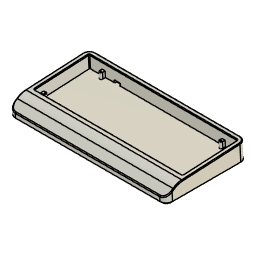
SK-Vault 37 (Autodesk Fusion 360 design; units mm, degrees)
Autodesk Fusion 360 part; units mm, degrees
sketch "Base Plane Sketch" plane through (0, 0, 0) normal (0, 0, 1) x (1, 0, 0)
  line L0 (0, 0) -> (209.55, 0) construction
  line L1 (209.55, 0) -> (209.55, -57.15) construction
  line L2 (28.575, -76.2) -> (180.975, -76.2) construction
  line L3 (-7.5, 7.5) -> (217.05, 7.5)
  line L4 (217.05, 7.5) -> (217.05, -64.65)
  line L5 (21.075, -83.7) -> (188.475, -83.7)
  line L6 (-7.5, 7.5) -> (-7.5, -64.65)
  line L7 (-7.5, -64.65) -> (-7.5, -83.7)
  line L8 (-7.5, -83.7) -> (21.075, -83.7)
  line L9 (188.475, -83.7) -> (217.05, -83.7)
  line L10 (217.05, -83.7) -> (217.05, -64.65)
  line L11 (-7.5, -83.7) -> (-7.5, -90.7)
  line L12 (-7.5, -90.7) -> (217.05, -90.7)
  line L13 (217.05, -90.7) -> (217.05, -83.7)
  line L14 (-1.075, 1.075) -> (-1.075, -57.15)
  line L15 (27.5, -77.275) -> (182.05, -77.275)
  line L16 (210.625, 1.075) -> (210.625, -58.225)
  line L17 (0, 1.075) -> (210.625, 1.075)
  line L18 (-1.075, -57.15) -> (-1.075, -58.225)
  line L19 (0, 1.075) -> (-1.075, 1.075)
  line L20 (209.55, 0) -> (190.5, 0) construction
  line L21 (190.5, 0) -> (190.5, -19.05) construction
  line L22 (190.5, -19.05) -> (209.55, -19.05) construction
  line L23 (209.55, -19.05) -> (209.55, 0) construction
  line L24 (190.5, -9.525) -> (209.55, -9.525) construction
  line L25 (200.025, -19.05) -> (200.025, 0) construction
  circle A0 centre (19.05, -2.525) radius 2.25
  line L26 (19.05, -2.525) -> (190.5, -2.525) construction
  circle A1 centre (190.5, -2.525) radius 2.25
  line L27 (21.3, -2.525) -> (21.3, 1.075)
  line L28 (192.75, -2.525) -> (192.75, 1.075)
  line L29 (188.25, -2.525) -> (188.25, 1.075)
  line L30 (16.8193, -2.2307) -> (16.8193, 1.075)
  line L31 (-1.075, -58.225) -> (-1.075, -77.275)
  line L32 (-1.075, -77.275) -> (27.5, -77.275)
  line L33 (210.625, -58.225) -> (210.625, -77.275)
  line L34 (210.625, -77.275) -> (182.05, -77.275)
  line L35 (-0.125, 0.125) -> (209.675, 0.125) construction
  line L36 (209.675, 0.125) -> (209.675, -76.325) construction
  line L37 (-0.125, -76.325) -> (-0.125, 0.125) construction
  line L38 (47.5, -76.325) -> (47.5, -57.275) construction
  line L39 (47.5, -57.275) -> (28.7, -57.275) construction
  line L40 (28.7, -57.275) -> (28.7, -76.325) construction
  line L41 (180.85, -76.325) -> (180.85, -57.275) construction
  line L42 (180.85, -57.275) -> (162.05, -57.275) construction
  line L43 (162.05, -57.275) -> (162.05, -76.325) construction
  circle A2 centre (19.05, -2.525) radius 1 construction
  circle A3 centre (190.5, -2.525) radius 1 construction
  circle A4 centre (207.284, -66.384) radius 1 construction
  circle A5 centre (2.266, -66.384) radius 1 construction
  line L44 (28.7, -76.325) -> (-0.125, -76.325) construction
  line L45 (209.675, -76.325) -> (180.85, -76.325) construction
  line L46 (162.05, -76.325) -> (47.5, -76.325) construction
  line L47 (179.9, -76.325) -> (179.9, -77.275)
  line L48 (163, -76.325) -> (163, -77.275)
  line L49 (29.65, -76.325) -> (29.65, -77.275)
  line L50 (46.55, -76.325) -> (46.55, -77.275)
  circle A6 centre (2.266, -66.384) radius 2.25
  circle A7 centre (207.284, -66.384) radius 2.25
  line L51 (207.284, -64.134) -> (210.625, -64.134)
  line L52 (207.284, -68.634) -> (210.625, -68.634)
  line L53 (2.266, -64.134) -> (-1.075, -64.134)
  line L54 (2.266, -68.634) -> (-1.075, -68.634)
  point P0 (9.525, -9.525)
  point P1 (9.525, -47.625)
  dimension "d1" = 209.55
  dimension "d2" = 57.15
  dimension "d39" = 7
  dimension "d117" = 19.05
  dimension "d118" = 19.05
  dimension "d122" = 4.5
  dimension "d180" = 209.8
  dimension "d181" = 76.45
  dimension "d182" = 19.05
  dimension "d183" = 18.8
  dimension "d184" = 28.825
  dimension "d185" = 18.8
  dimension "d186" = 19.05
  dimension "d187" = 28.825
  dimension "d188" = 2
  dimension "d189" = 2
  dimension "d190" = 2
  dimension "d191" = 2
  dimension "d192" = 19.175
  dimension "d193" = 2.65
  dimension "d194" = 2.65
  dimension "d195" = 19.175
  dimension "d196" = 2.391
  dimension "d197" = 9.941
  dimension "d198" = 9.941
  dimension "d199" = 2.391
  dimension "d202" = 4.5
  dimension "d203" = 4.5
  constraint coincident L0.start origin
  constraint horizontal L0
  constraint perpendicular L0 L1
  constraint perpendicular L5 L7
  constraint perpendicular L4 L9
  constraint vertical L11
  constraint perpendicular L10 L12
  constraint perpendicular L9 L13
  constraint perpendicular L14 L19
  constraint horizontal L20
  constraint vertical L21
  constraint horizontal L22
  constraint vertical L23
  constraint midpoint L21 L24.start
  constraint midpoint L23 L24.end
  constraint midpoint L22 L25.start
  constraint midpoint L20 L25.end
  constraint coincident A0.centre L26.start
  constraint coincident L21 L26.end
  constraint perpendicular L21 L26
  constraint coincident L26.end A1.centre
  constraint coincident A0 L27.start
  constraint coincident L26 L27.start
  constraint coincident L17 L27.end
  constraint tangent A0 L27
  constraint coincident A1 L28.start
  constraint coincident L17 L28.end
  constraint tangent A1 L28
  constraint perpendicular L17 L28
  constraint coincident L26 L29.start
  constraint coincident A1 L29.start
  constraint coincident L17 L29.end
  constraint tangent A1 L29
  constraint coincident A0 L30.start
  constraint coincident L17 L30.end
  constraint perpendicular L17 L30
  constraint equal A0 A1
  constraint perpendicular L15 L31
  constraint perpendicular L31 L32
  constraint perpendicular L15 L33
  constraint horizontal L35
  constraint vertical L36
  constraint horizontal L45
  constraint vertical L37
  constraint vertical L38
  constraint horizontal L39
  constraint vertical L40
  constraint coincident L40.end L45
  constraint vertical L41
  constraint horizontal L42
  constraint vertical L43
  constraint coincident L43.end L45
  constraint collinear L44 L45
  constraint collinear L45 L46
  constraint coincident L15 L47.end
  constraint perpendicular L15 L47
  constraint coincident L15 L48.end
  constraint perpendicular L15 L48
  constraint coincident L15 L49.end
  constraint perpendicular L15 L49
  constraint coincident L15 L50.end
  constraint perpendicular L15 L50
  constraint concentric A5 A6
  constraint concentric A4 A7
  constraint coincident A7 L51.start
  constraint coincident L33 L51.end
  constraint tangent A7 L51
  constraint perpendicular L33 L51
  constraint coincident A7 L52.start
  constraint coincident L33 L52.end
  constraint tangent A7 L52
  constraint perpendicular L33 L52
  constraint coincident A6 L53.start
  constraint coincident L31 L53.end
  constraint tangent A6 L53
  constraint perpendicular L31 L53
  constraint coincident A6 L54.start
  constraint coincident L31 L54.end
  constraint tangent A6 L54
  constraint perpendicular L31 L54
  measures "d1" distance of L0.start L0.end
  measures "d2" distance of L0.end L1.end
  measures "d39" distance of L7.end L11.end
  measures "d117" distance of L0.end L20.end
  measures "d118" distance of L0.end L22.end
  measures "d122" diameter of A0
  measures "d180" distance of L35.start L35.end
  measures "d181" distance of L35.start L37.start
  measures "d182" distance of L40.end L39.end
  measures "d183" distance of L38.end L39.end
  measures "d184" distance of L37 L40
  measures "d185" distance of L43.end L41.start
  measures "d186" distance of L43.end L42.end
  measures "d187" distance of L36 L41
  measures "d188" diameter of A2
  measures "d189" diameter of A3
  measures "d190" diameter of A4
  measures "d191" diameter of A5
  measures "d192" distance of L37 A0.centre
  measures "d193" distance of L35 A0.centre
  measures "d194" distance of L35 L26.end
  measures "d195" distance of L36 L26.end
  measures "d196" distance of L37 A5.centre
  measures "d197" distance of A5.centre L45
  measures "d198" distance of A4.centre L45
  measures "d199" distance of L36 A4.centre
  measures "d202" diameter of A6
  measures "d203" diameter of A7
extrude "External Base Extrude" add sketch "Base Plane Sketch" along normal blind 21.06
extrude "Internal Base Extrude" add sketch "Base Plane Sketch" 1 faces at (85.3667, -86.225, 0) along normal blind 3 contours L14 L15 L16 L17 L18 L19 A0 A1 L27 L28 L29 L30 L31 L32 L33 L34 A6 A7 L51 L52 L53 L54 | L17 A0 L27 L30 | L31 A6 L53 L54 | A0 | A6 | L17 A1 L28 L29 | A1 | L33 A7 L51 L52 | A7
sketch "Side Plane Sketch" plane through (-7.5, 0, 0) normal (-1, 0, 0) x (0, -1, 0)
  line L0 (90.7, 0) -> (90.7, 21.06)
  line L1 (90.7, 21.06) -> (-7.5, 21.06)
  line L2 (-7.5, 21.06) -> (-7.5, 0)
  line L3 (-7.5, 0) -> (90.7, 0)
  line L4 (90.7, 21.06) -> (107.8598, 10)
  line L5 (107.8598, 10) -> (107.8598, 0)
  line L6 (107.8598, 0) -> (90.7, 0)
  dimension "d149" = 10
  constraint coincident L0.end L1.start
  constraint perpendicular L3 L5
  constraint coincident L0.start L3.end
  constraint perpendicular L0 L6
  measures "d149" distance of L4.end L5.end
extrude "Wrist Wrest Extrude" add sketch "Side Plane Sketch" against normal up to surface (224.55 mm away) contours L0 L4 L5 L6
fillet "Outside Vertical Fillets" radius 9 4 edges at (-7.5, -107.8598, 5) (217.05, -107.8598, 5) (217.05, 7.5, 10.53) (-7.5, 7.5, 10.53)
fillet "Wrist Wrest Angle Fillet" radius 23.5 1 edges at (104.775, -90.7, 21.06)
fillet "Inside Case Vertical Fillets" radius 1 4 edges at (210.625, 1.075, 12.03) (210.625, -77.275, 12.03) (-1.075, -77.275, 12.03) (-1.075, 1.075, 12.03)
chamfer "Top Outside Edge Chamfer" distance 1 angle 45 12 edges at (-7.5, -42.6415, 21.06) (-7.5, -90.4185, 20.1037) (-7.5, -97.6869, 16.5567) (-4.864, -105.2238, 11.699) (104.775, -107.8598, 10) (214.414, -105.2238, 11.699) (217.05, -97.6869, 16.5567) (217.05, -90.4185, 20.1037) (217.05, -42.6415, 21.06) (214.414, 4.864, 21.06) (104.775, 7.5, 21.06) (-4.864, 4.864, 21.06)
chamfer "Top Inside Edge Chamfer" distance 1 angle 45 8 edges at (210.625, -38.1, 21.06) (210.3321, -76.9821, 21.06) (104.775, -77.275, 21.06) (-0.7821, -76.9821, 21.06) (-1.075, -38.1, 21.06) (-0.7821, 0.7821, 21.06) (104.775, 1.075, 21.06) (210.3321, 0.7821, 21.06)
sketch "USB C Hole Internal" plane through (0, 1.075, 0) normal (0, -1, 0) x (1, 0, 0)
  line L0 (193, 10.9) -> (193, 3)
  line L1 (193, 3) -> (209.05, 3)
  line L2 (209.05, 3) -> (209.05, 17.06)
  line L3 (209.05, 17.06) -> (0.5, 17.06)
  line L4 (0.5, 17.06) -> (0.5, 3)
  line L5 (0.5, 3) -> (16.55, 3)
  line L6 (16.55, 3) -> (16.55, 10.9)
  line L7 (16.55, 10.9) -> (21.55, 10.9)
  line L8 (21.55, 10.9) -> (21.55, 3)
  line L9 (21.55, 3) -> (188, 3)
  line L10 (188, 3) -> (188, 10.9)
  line L11 (188, 10.9) -> (193, 10.9)
  line L12 (0.5, 3) -> (0, 3) construction
  line L13 (34.925, 3) -> (38.1, 3) construction
  line L14 (41.275, 6.66) -> (34.925, 6.66)
  line L15 (33.375, 5.11) -> (33.375, 4.55)
  line L16 (33.375, 3) -> (41.275, 3)
  line L17 (42.825, 4.55) -> (42.825, 5.11)
  line L18 (42.825, 6.66) -> (33.375, 3) construction
  line L19 (33.375, 6.66) -> (42.825, 3) construction
  arc A0 (34.925, 6.66) -> (33.375, 5.11) centre (34.925, 5.11) ccw
  arc A1 (42.825, 5.11) -> (41.275, 6.66) centre (41.275, 5.11) ccw
  arc A2 (41.275, 3) -> (42.825, 4.55) centre (41.275, 4.55) ccw
  arc A3 (33.375, 4.55) -> (34.925, 3) centre (34.925, 4.55) ccw
  line L20 (209.625, 20.06) -> (-0.075, 20.06)
  line L21 (-0.075, 20.06) -> (-0.075, 3)
  line L22 (-0.075, 3) -> (209.625, 3)
  line L23 (209.625, 3) -> (209.625, 20.06)
  point P0 (38.1, 4.83)
  dimension "d75" = 0.5
  dimension "d79" = 1.55
  dimension "d80" = 9.45
  dimension "d82" = 38.1
  dimension "d83" = 3.66
  constraint coincident L4.end L5.start
  constraint perpendicular L4 L12
  constraint parallel L5 L13
  constraint horizontal L14
  constraint perpendicular L14 L15
  constraint parallel L14 L16
  constraint parallel L15 L17
  constraint coincident L18 P0
  constraint coincident L19 P0
  constraint coincident L19.start L15
  constraint coincident L19.start L14
  constraint tangent L15 A0
  constraint tangent L14 A0
  constraint coincident L18.start L14
  constraint coincident L18.start L17
  constraint tangent L14 A1
  constraint tangent L17 A1
  constraint equal A0 A1
  constraint coincident L19.end L17
  constraint coincident L19.end L16
  constraint tangent L17 A2
  constraint tangent L16 A2
  constraint equal A0 A2
  constraint coincident L12.end L13
  constraint coincident L16.start L15
  constraint tangent L13 A3
  constraint tangent L15 A3
  constraint equal A0 A3
  measures "d75" distance of L4.end L12.end
  measures "d79" radius of A0
  measures "d80" distance of L15 L17
  measures "d82" distance of L12.end L13.end
  measures "d83" distance of L13.end L14
extrude "Internal USB C Extrude Cut" cut sketch "USB C Hole Internal" against normal blind 24 contours L9 L14 L15 L16 L17 A0 A1 A2 A3 L22
sketch "USB C Hole External" plane through (0, 7.5, 0) normal (0, 1, 0) x (-1, 0, 0)
  arc A0 (-42.825, 4.55) -> (-41.275, 3) centre (-41.275, 4.55) ccw
  line L0 (-42.825, 4.55) -> (-42.825, 5.11)
  arc A1 (-41.275, 6.66) -> (-42.825, 5.11) centre (-41.275, 5.11) ccw
  line L1 (-41.275, 6.66) -> (-34.925, 6.66)
  arc A2 (-33.375, 5.11) -> (-34.925, 6.66) centre (-34.925, 5.11) ccw
  line L2 (-33.375, 5.11) -> (-33.375, 4.55)
  arc A3 (-34.925, 3) -> (-33.375, 4.55) centre (-34.925, 4.55) ccw
  line L3 (-42.825, 4.83) -> (-33.375, 4.83) construction
  line L4 (-38.1, 6.66) -> (-38.1, 3) construction
  line L5 (-34.925, 8.91) -> (-41.275, 8.91)
  line L6 (-45.075, 5.11) -> (-45.075, 4.55)
  line L7 (-41.275, 0.75) -> (-34.925, 0.75)
  line L8 (-31.125, 4.55) -> (-31.125, 5.11)
  line L9 (-31.125, 8.91) -> (-45.075, 0.75) construction
  line L10 (-45.075, 8.91) -> (-31.125, 0.75) construction
  arc A4 (-41.275, 8.91) -> (-45.075, 5.11) centre (-41.275, 5.11) ccw
  arc A5 (-31.125, 5.11) -> (-34.925, 8.91) centre (-34.925, 5.11) ccw
  arc A6 (-34.925, 0.75) -> (-31.125, 4.55) centre (-34.925, 4.55) ccw
  arc A7 (-45.075, 4.55) -> (-41.275, 0.75) centre (-41.275, 4.55) ccw
  line L11 (-1.5, 0) -> (-1.5, 20.06)
  line L12 (-208.05, 20.06) -> (-208.05, 0)
  line L13 (-1.5, 20.06) -> (-208.05, 20.06)
  line L14 (-34.925, 3) -> (-41.275, 3)
  line L15 (-208.05, 0) -> (-1.5, 0)
  point P0 (-38.1, 4.83)
  dimension "d86" = 13.95
  dimension "d87" = 8.16
  dimension "d88" = 3.8
  constraint midpoint L0 L3.start
  constraint midpoint L2 L3.end
  constraint midpoint L1 L4.start
  constraint horizontal L5
  constraint perpendicular L5 L6
  constraint parallel L5 L7
  constraint parallel L6 L8
  constraint coincident L9 P0
  constraint coincident L10 P0
  constraint midpoint L3 P0
  constraint coincident L10.start L6
  constraint coincident L10.start L5
  constraint tangent L6 A4
  constraint tangent L5 A4
  constraint coincident L9.start L5
  constraint coincident L9.start L8
  constraint tangent L5 A5
  constraint tangent L8 A5
  constraint equal A4 A5
  constraint coincident L10.end L8
  constraint coincident L10.end L7
  constraint tangent L8 A6
  constraint tangent L7 A6
  constraint equal A4 A6
  constraint coincident L9.end L7
  constraint coincident L9.end L6
  constraint tangent L7 A7
  constraint tangent L6 A7
  constraint equal A4 A7
  measures "d86" distance of L9.end L10.end
  measures "d87" distance of L10.start L9.end
  measures "d88" radius of A4
extrude "External USB C Extrude Cut" cut sketch "USB C Hole External" against normal blind 4 contours A0 L0 A1 L1 A2 L2 A3 L14 | L5 L6 L7 L8 A4 A5 A6 A7
ref_plane "WorkPlane2" through (104.775, -107.8598, 0) normal (0, 0.052336, 0.99863) x (1, 0, 0)
extrude "Extrude18" add 1 faces at (70.35, -69.4065, 0) along direction (0, 0, -1) up to surface end surface through (104.775, -107.8598, 0) normal (0, 0.052336, 0.99863) offset 0
chamfer "Chamfer9" distance 3 angle 45 8 edges at (217.05, -50.1799, -3.0229) (214.414, -105.2238, -0.1381) (104.775, -107.8598, 0) (-4.864, -105.2238, -0.1381) (-7.5, -50.1799, -3.0229) (-4.864, 4.864, -5.9076) (104.775, 7.5, -6.0458) (214.414, 4.864, -5.9076)
extrude "Screw Post Extrude" add sketch "Base Plane Sketch" along normal blind 8.41 from surface at 3 contours L17 A0 L27 L30 | L31 A6 L53 L54 | A0 | A6 | L17 A1 L28 L29 | A1 | L33 A7 L51 L52 | A7
hole "Top Left Screw Hole" at (19.05, -2.525, 11.41) direction (0, 0, -1) diameter 1.8 depth 4 tip angle 180
hole "Top Right Screw Hole" at (190.5, -2.525, 11.41) direction (0, 0, -1) diameter 1.8 depth 4 tip angle 180
hole "Bottom Right Screw Hole" at (207.284, -66.384, 11.41) direction (0, 0, -1) diameter 1.8 depth 4 tip angle 180
hole "Bottom Left Screw Hole" at (2.266, -66.384, 11.41) direction (0, 0, -1) diameter 1.8 depth 4 tip angle 180
move_body "Rotate Case" bodies 1 to x (1, 0, 0) y (0, 0.99863, 0.052336) z (0, -0.052336, 0.99863) at (0, 0.0092, 5.6491)
equation "d10 = 18.06 mm + 3 mm"
equation "d130 = 7.9 mm + 0.51 mm"
